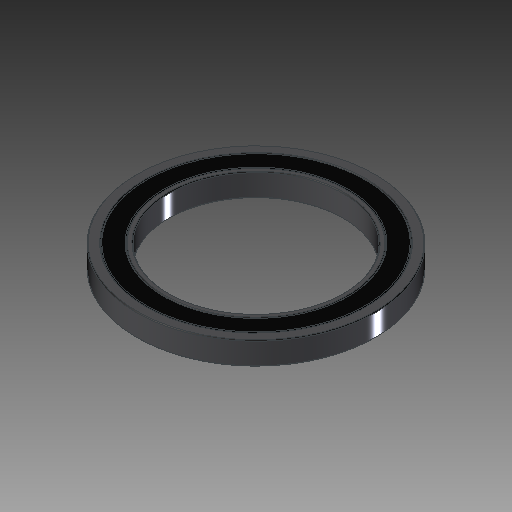
# Autodesk Inventor part: 2123_Bearing_V1
Saved by Autodesk Inventor 2020 (Build 240168000, 168)
## iProperties
Created: 2017-06-14
Part Number: 2123_Bearing_V1
Material: Iron, Cast
Document SubType Name: Modeling
Designer: MPI
Density: 7.15 g/cm^3
Appearance: Iron Gray
Mass: 971.838 g
Surface Area: 544.816 cm^2
Volume: 135.921 cm^3
Author: MPI
Autodesk Inventor part; units mm, degrees
ref_plane "YZ Plane" through (0, 0, 0) normal (1, 0, 0) x (0, 1, 0)
ref_plane "XZ Plane" through (0, 0, 0) normal (0, 1, 0) x (-1, 0, 0)
ref_plane "XY Plane" through (0, 0, 0) normal (0, 0, 1) x (1, 0, 0)
sketch "Sketch1" plane through (0, 0, 0) normal (0, 1, 0) x (-1, 0, 0)
  circle A0 centre (0, 0) radius 57.15
  circle A1 centre (0, 0) radius 78.4987
  circle A2 centre (0, 0) radius 72.1487
  circle A3 centre (0, 0) radius 60.325
  dimension "d0" = 114.3
  dimension "d1" = 156.9974
  dimension "d2" = 6.35
  dimension "d3" = 3.175
  constraints: 4 centre point, 2 coincident
  measures "d0" diameter of A0
  measures "d1" diameter of A1
  measures "d2" radial gap between concentric circles of A1 A2
  measures "d3" radial gap between concentric circles of A0 A3
extrude "Extrusion1" add sketch "Sketch1" along normal mid plane 15.0114 contours A1
sketch "Sketch2" plane through (0, 0, 0) normal (0, 1, 0) x (-1, 0, 0)
  circle A0 centre (0, 0) radius 57.15
  circle A1 centre (0, 0) radius 78.4987
  circle A2 centre (0, 0) radius 72.1487
  circle A3 centre (0, 0) radius 60.325
  dimension "d6" = 114.3
  dimension "d7" = 156.9974
  dimension "d8" = 6.35
  dimension "d9" = 3.175
  constraints: 4 centre point, 2 coincident
  measures "d6" diameter of A0
  measures "d7" diameter of A1
  measures "d8" radial gap between concentric circles of A1 A2
  measures "d9" radial gap between concentric circles of A0 A3
extrude "Extrusion2" add sketch "Sketch2" along normal mid plane 15.0114 separate body contours A2
sketch "Sketch3" plane through (0, 0, 0) normal (0, 1, 0) x (-1, 0, 0)
  circle A0 centre (0, 0) radius 57.15
  circle A1 centre (0, 0) radius 78.4987
  circle A2 centre (0, 0) radius 72.1487
  circle A3 centre (0, 0) radius 60.325
  dimension "d16" = 15.0114
  dimension "d12" = 114.3
  dimension "d13" = 156.9974
  dimension "d14" = 6.35
  dimension "d15" = 3.175
  constraints: 4 centre point, 2 coincident
  measures "d12" diameter of A0
  measures "d13" diameter of A1
  measures "d14" radial gap between concentric circles of A1 A2
  measures "d15" radial gap between concentric circles of A0 A3
extrude "Extrusion3" add sketch "Sketch3" along normal mid plane 15.0114 separate body contours A3
chamfer "Chamfer1" distance 0.508 angle 45 8 edges at (78.4987, 7.5057, 0) (78.4987, -7.5057, 0) (72.1487, 7.5057, 0) (72.1487, -7.5057, 0) (60.325, 7.5057, 0) (60.325, -7.5057, 0) (57.15, 7.5057, 0) (57.15, -7.5057, 0)
body "Solid1"
body "Solid2"
body "Solid3"
